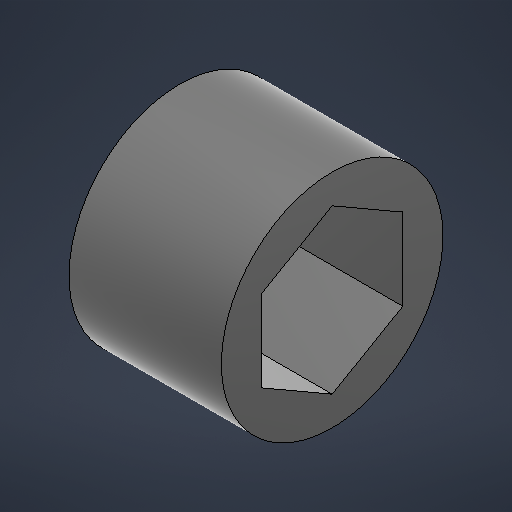
# Autodesk Inventor part: 3DPRINT,KICKER,MOTOR,SUPPORT-PLATE,SPACER
Saved by Autodesk Inventor 2026.1 (Build 301233020, 233B)
## iProperties
Created: 2026-02-14
Part Number: 3DPRINT,KICKER,MOTOR,SUPPORT-PLATE,SPACER
Material: ABS Plastic
Document SubType Name: Modeling
Designer: Owen L
Density: 1.06 g/cm^3
Appearance: Smooth - Black
Author: Owen L
Autodesk Inventor part; units mm, degrees
ref_plane "YZ Plane" through (0, 0, 0) normal (1, 0, 0) x (0, 1, 0)
ref_plane "XZ Plane" through (0, 0, 0) normal (0, 1, 0) x (-1, 0, 0)
ref_plane "XY Plane" through (0, 0, 0) normal (0, 0, 1) x (1, 0, 0)
sketch "Sketch1" plane through (0, 0, 0) normal (1, 0, 0) x (0, 1, 0)
  line L0 (3.7395, -6.477) -> (-3.7395, -6.477)
  line L1 (-3.7395, -6.477) -> (-7.479, 0)
  line L2 (-7.479, 0) -> (-3.7395, 6.477)
  line L3 (-3.7395, 6.477) -> (3.7395, 6.477)
  line L4 (3.7395, 6.477) -> (7.479, 0)
  line L5 (7.479, 0) -> (3.7395, -6.477)
  circle A0 centre (0, 0) radius 10.16
  dimension "d0" = 20.32
  dimension "d1" = 12.954
  constraints: 12 end point, 2 coincident, 1 centre point, 1 horizontal, 13 other
  measures "d0" diameter of A0
  measures "d1" distance between parallel lines of L0 L3
extrude "Extrusion1" add sketch "Sketch1" along normal blind 13.969
body "Solid1"
